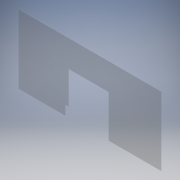
# Autodesk Inventor part: Long Wall
Saved by Autodesk Inventor 2017 (Build 210142000, 142)
## iProperties
Created: 2017-01-16
Part Number: Long Wall
Material: Polycarbonate, Clear
Document SubType Name: Modeling
Designer: Ben
Density: 1.2 g/cm^3
Appearance: Polycarbonate - Clear
Mass: 566.199 g
Surface Area: 5980.63 cm^2
Volume: 471.832 cm^3
Author: Ben
Autodesk Inventor part; units mm, degrees
ref_plane "YZ Plane" through (0, 0, 0) normal (1, 0, 0) x (0, 1, 0)
ref_plane "XZ Plane" through (0, 0, 0) normal (0, 1, 0) x (-1, 0, 0)
ref_plane "XY Plane" through (0, 0, 0) normal (0, 0, 1) x (1, 0, 0)
sketch "Sketch1" plane through (0, 0, 0) normal (0, 0, 1) x (1, 0, 0)
  line L0 (0, 0) -> (247.65, 0)
  line L1 (762, 0) -> (762, 368.3)
  line L2 (762, 368.3) -> (0, 368.3)
  line L3 (0, 368.3) -> (0, 0)
  line L4 (752.475, 368.3) -> (752.475, 0) construction
  line L5 (762, 184.15) -> (0, 184.15) construction
  line L6 (381, 368.3) -> (381, 0) construction
  line L7 (762, 238.125) -> (0, 238.125) construction
  circle A0 centre (381, 238.125) radius 1.5875
  circle A1 centre (295.275, 238.125) radius 1.5875
  circle A2 centre (209.55, 238.125) radius 1.5875
  circle A3 centre (123.825, 238.125) radius 1.5875
  circle A4 centre (38.1, 238.125) radius 1.5875
  circle A5 centre (466.725, 238.125) radius 1.5875
  circle A6 centre (552.45, 238.125) radius 1.5875
  circle A7 centre (638.175, 238.125) radius 1.5875
  circle A8 centre (723.9, 238.125) radius 1.5875
  circle A9 centre (752.475, 184.15) radius 1.5875
  circle A10 centre (752.475, 107.95) radius 1.5875
  circle A11 centre (752.475, 31.75) radius 1.5875
  circle A12 centre (752.475, 260.35) radius 1.5875
  circle A13 centre (752.475, 184.15) radius 1.5875
  circle A14 centre (752.475, 107.95) radius 1.5875
  circle A15 centre (752.475, 336.55) radius 1.5875
  circle A16 centre (752.475, 260.35) radius 1.5875
  circle A17 centre (752.475, 184.15) radius 1.5875
  line L8 (9.525, 368.3) -> (9.525, 0) construction
  circle A18 centre (9.525, 184.15) radius 1.5875
  circle A19 centre (9.525, 107.95) radius 1.5875
  circle A20 centre (9.525, 31.75) radius 1.5875
  circle A21 centre (9.525, 260.35) radius 1.5875
  circle A22 centre (9.525, 184.15) radius 1.5875
  circle A23 centre (9.525, 107.95) radius 1.5875
  circle A24 centre (9.525, 336.55) radius 1.5875
  circle A25 centre (9.525, 260.35) radius 1.5875
  circle A26 centre (9.525, 184.15) radius 1.5875
  line L9 (482.6, 0) -> (482.6, 228.6)
  line L10 (482.6, 228.6) -> (266.7, 228.6)
  line L11 (266.7, 228.6) -> (266.7, 50.8)
  line L12 (482.6, 0) -> (762, 0)
  line L13 (266.7, 0) -> (482.6, 0) construction
  line L14 (266.7, 50.8) -> (247.65, 50.8)
  line L15 (247.65, 50.8) -> (247.65, 0)
  line L16 (266.7, 50.8) -> (266.7, 0) construction
  line L17 (247.65, 0) -> (266.7, 0) construction
  dimension "d0" = 762
  dimension "d1" = 368.3
  dimension "d12" = 9.525
  dimension "d16" = 85.725
  dimension "d23" = 85.725
  dimension "d28" = 3.175
  dimension "d31" = 76.2
  dimension "d34" = 76.2
  dimension "d39" = 9.525
  dimension "d41" = 101.6
  dimension "d42" = 114.3
  dimension "d43" = 19.05
  dimension "d44" = 50.8
  dimension "d45" = 44.45
  constraints: 36 end point, 27 centre point, 16 perpendicular, 11 symmetric about line, 7 horizontal, 6 midpoint, 6 parallel, 6 point on line, 3 vertical, 1 equal radius, 41 other
  measures "d0" distance of L0.start L1.start
  measures "d1" distance of L2.end L0.start
  measures "d12" distance between parallel lines of L4 L1
  measures "d16" distance of A0.centre A1.centre
  measures "d23" distance of A0.centre A5.centre
  measures "d28" diameter of A8
  measures "d31" distance of A9.centre A10.centre
  measures "d34" distance of A9.centre A12.centre
  measures "d39" distance between parallel lines of L7 L10
  measures "d41" distance between parallel lines of L6 L9
  measures "d42" distance between parallel lines of L11 L6
  measures "d43" distance of L11.end L14.end
  measures "d44" distance of L14.end L0.end
  measures "d45" distance between parallel lines of L5 L10
extrude "Extrusion1" add sketch "Sketch1" along normal blind 1.5875
body "Solid1"
